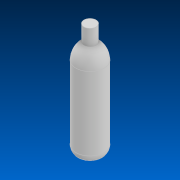
# Autodesk Inventor part: CO2Cartridge16g
Saved by Autodesk Inventor 2020.4 (Build 244396010, 396A)
## iProperties
Created: 2022-09-12
Part Number: CO2Cartridge16g
Material: Generic
Document SubType Name: Modeling
Designer: Val
Density: 1 g/cm^3
Appearance: Default
Author: Val
Autodesk Inventor part; units mm, degrees
ref_plane "YZ Plane" through (0, 0, 0) normal (1, 0, 0) x (0, 1, 0)
ref_plane "XZ Plane" through (0, 0, 0) normal (0, 1, 0) x (-1, 0, 0)
ref_plane "XY Plane" through (0, 0, 0) normal (0, 0, 1) x (1, 0, 0)
sketch "Sketch1" plane through (0, 0, 0) normal (0, 0, 1) x (1, 0, 0)
  line L0 (10.85, 64) -> (10.85, 6)
  line L1 (10.85, 64) -> (0, 64)
  line L2 (0, 64) -> (0, 6)
  line L3 (0, 6) -> (10.85, 6)
  line L4 (0, 64) -> (0, 76)
  line L5 (0, 76) -> (4.65, 76)
  arc A0 (10.85, 64) -> (4.65, 76) centre (-3.8629, 64) ccw
  line L6 (4.65, 76) -> (0, 76)
  line L7 (0, 76) -> (0, 88.2)
  line L8 (0, 88.2) -> (4.65, 88.2)
  line L9 (4.65, 88.2) -> (4.65, 76)
  line L10 (0, 6) -> (0, 0)
  arc A1 (0, 0) -> (10.85, 6) centre (0, 12.8102) ccw
  line L11 (0, 0) -> (10.85, 0)
  line L12 (10.85, 0) -> (10.85, 6)
  dimension "d0" = 58
  dimension "d1" = 10.85
  dimension "d2" = 12
  dimension "d3" = 4.65
  dimension "d4" = 12.2
  dimension "d5" = 6
  constraints: 26 end point, 4 horizontal, 4 point on circle, 4 vertical, 3 perpendicular, 2 centre point, 2 parallel, 2 tangent, 1 coincident, 1 collinear
  measures "d0" distance of L0.start L0.end
  measures "d1" distance of L0.start L1.end
  measures "d2" distance of L1.end L4.end
  measures "d3" distance of L4.end L5.end
  measures "d4" distance of L8.end L5.end
  measures "d5" distance of L2.end L10.end
revolve "Revolution1" add sketch "Sketch1" angle 360 about axis through (0, 64, 0) along (0, -1, 0) contours L0 L3 L2 L1 | L1 L4 L5 A0 | A1 L10 L3 | L5 L7 L8 L9
fillet "Fillet1" radius 6 1 edges at (-10.85, 6, 0)
body "Solid1"
